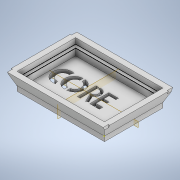
# Autodesk Inventor part: Rack holder aluminium
Saved by Autodesk Inventor 2021 (Build 250183000, 183)
## iProperties
Created: 2021-05-21
Part Number: Rack holder aluminium
Material: Generic
Document SubType Name: Modeling
Designer: Olivi
Density: 1 g/cm^3
Appearance: Default
Author: Olivi
Autodesk Inventor part; units mm, degrees
ref_plane "YZ Plane" through (0, 0, 0) normal (1, 0, 0) x (0, 1, 0)
ref_plane "XZ Plane" through (0, 0, 0) normal (0, 1, 0) x (-1, 0, 0)
ref_plane "XY Plane" through (0, 0, 0) normal (0, 0, 1) x (1, 0, 0)
sketch "Sketch1" plane through (0, 0, 0) normal (0, 1, 0) x (-1, 0, 0)
  line L0 (0, 0) -> (0, -85.5)
  line L1 (0, -85.5) -> (127.8, -85.5)
  line L2 (127.8, -85.5) -> (127.8, 0)
  line L3 (127.8, 0) -> (0, 0)
  dimension "d0" = 85.5
  dimension "d1" = 127.8
  constraints: 8 end point, 3 perpendicular, 1 vertical
  measures "d0" distance of L0.start L0.end
  measures "d1" distance of L0.end L1.end
extrude "Extrusion2" add sketch "Sketch1" along normal blind 7
sketch "Sketch3" plane through (0, 7, 0) normal (0, 1, 0) x (1, 0, 0)
  point P0 (0, 0)
sketch "Sketch4" plane through (0, 7, 0) normal (0, 1, 0) x (1, 0, 0)
  arc A0 (-101.824, 57.4968) -> (-102.1452, 30.5151) centre (-105.5468, 44.0484) ccw
  arc A1 (-103.7513, 52.0362) -> (-103.7513, 35.012) centre (-104.5875, 43.5241) ccw
  line L0 (-103.7513, 52.0362) -> (-101.824, 57.4968)
  line L1 (-103.7513, 35.012) -> (-102.1452, 30.5151)
  arc A2 (-88.634, 52.8416) -> (-88.8908, 35.2488) centre (-87.1081, 44.021) ccw
  arc A3 (-85.3254, 35.2488) -> (-85.5822, 52.8416) centre (-87.1081, 44.021) ccw
  arc A4 (-85.5822, 30.5151) -> (-85.5822, 57.4968) centre (-86.7037, 44.006) ccw
  line L2 (-85.5822, 57.4968) -> (-85.5822, 52.8416)
  line L3 (-85.3254, 35.2488) -> (-85.5822, 30.5151)
  line L4 (-88.8908, 35.2488) -> (-88.8908, 30.2611)
  line L5 (-88.634, 57.4969) -> (-88.634, 52.8416)
  arc A5 (-88.634, 57.4969) -> (-88.8908, 30.2611) centre (-88.5011, 43.8765) ccw
  line L6 (-69.8, 57.4969) -> (-69.8, 30.2611)
  line L7 (-69.8, 30.2611) -> (-65.8, 30.2611)
  line L8 (-65.8, 30.2611) -> (-65.8, 57.4969)
  line L9 (-65.8, 57.4969) -> (-69.8, 57.4969)
  line L10 (-57.9844, 30.2611) -> (-64.357, 43.879)
  arc A6 (-64.357, 43.879) -> (-64.357, 55.1692) centre (-63.6585, 49.5241) ccw
  line L11 (-57.9844, 30.2611) -> (-54.5512, 31.8677)
  line L12 (-54.5512, 31.8677) -> (-59.1663, 41.7297)
  arc A7 (-59.1663, 41.7297) -> (-64.357, 57.4969) centre (-62.8, 49.2714) ccw
  line L13 (-64.357, 57.4969) -> (-64.357, 55.1692)
  line L14 (-51.8, 58.0868) -> (-51.8, 30.2611)
  line L15 (-51.8, 30.2611) -> (-37.8, 30.2611)
  line L16 (-37.8, 30.2611) -> (-37.8, 35.2488)
  line L17 (-37.8, 35.2488) -> (-47.8, 35.2488)
  line L18 (-47.8, 35.2488) -> (-47.8, 43.5)
  line L19 (-47.8, 43.5) -> (-39.7884, 43.5)
  line L20 (-39.7884, 43.5) -> (-39.7884, 46.5)
  line L21 (-39.7884, 46.5) -> (-47.8, 46.5)
  line L22 (-47.8, 46.5) -> (-47.8, 54.5)
  line L23 (-47.8, 54.5) -> (-37.8, 54.5)
  line L24 (-37.8, 54.5) -> (-37.8, 58.0868)
  line L25 (-37.8, 58.0868) -> (-51.8, 58.0868)
  line L26 (-127.8, 85.5) -> (-127.8, 0) projected
  line L27 (0, 85.5) -> (-127.8, 85.5) projected
  point P0 (0, 0)
  dimension "d28" = 62
  dimension "d29" = 65
  dimension "d30" = 76
  dimension "d31" = 80
  dimension "d32" = 90
  dimension "d35" = 27.4132
  dimension "d36" = 31
  dimension "d37" = 39
  dimension "d38" = 42
  dimension "d39" = 50.2512
  dimension "d40" = 22.2532
  dimension "d43" = 58
  constraints: 52 end point, 19 point on circle, 13 perpendicular, 8 centre point, 6 vertical, 5 point on line, 1 concentric
  measures "d28" distance between parallel lines of L26 L8
  measures "d29" distance from line of L26 A7.centre
  measures "d30" distance between parallel lines of L26 L14
  measures "d31" distance between parallel lines of L26 L22
  measures "d32" distance between parallel lines of L26 L24
  measures "d35" distance between parallel lines of L27 L25
  measures "d36" distance between parallel lines of L23 L27
  measures "d37" distance between parallel lines of L21 L27
  measures "d38" distance between parallel lines of L27 L19
  measures "d39" distance between parallel lines of L17 L27
  measures "d40" distance from line of L26 A0.centre
  measures "d43" distance between parallel lines of L26 L6
extrude "Extrusion3" cut sketch "Sketch4" against normal through all
sketch "Sketch5" plane through (0, 7, 0) normal (0, 1, 0) x (1, 0, 0)
  line L0 (-127.8, 0) -> (0, 0) projected
  line L1 (-127.8, 0) -> (0, 0)
  line L2 (0, 0) -> (0, 85.5) projected
  line L3 (0, 0) -> (0, 85.5)
  line L4 (0, 85.5) -> (-127.8, 85.5) projected
  line L5 (0, 85.5) -> (-127.8, 85.5)
  line L6 (-127.8, 85.5) -> (-127.8, 0)
  line L7 (-122.8, 80.5) -> (-5, 80.5)
  line L8 (-5, 80.5) -> (-5, 4.1226)
  line L9 (-5, 4.1226) -> (-122.8, 4.1226)
  line L10 (-122.8, 4.1226) -> (-122.8, 80.5)
  line L11 (-127.8, 85.5) -> (-127.8, 0) projected
  dimension "d44" = 5
  dimension "d45" = 5
  dimension "d46" = 5
  constraints: 16 end point, 5 perpendicular, 3 equal length
  measures "d44" distance between parallel lines of L2 L8
  measures "d45" distance between parallel lines of L6 L10
  measures "d46" distance between parallel lines of L4 L7
extrude "Extrusion4" add sketch "Sketch5" along normal blind 10
sketch "Sketch9" plane through (0, 17, 0) normal (0, 1, 0) x (1, 0, 0)
  line L0 (-127.8, 85.5) -> (-127.8, 0) projected
  line L1 (-127.8, 0) -> (-127.8, 85.5)
  line L2 (-127.8, 85.5) -> (0, 85.5)
  line L3 (0, 85.5) -> (0, 0)
  line L4 (0, 0) -> (-127.8, 0)
  line L5 (-122.8, 4.1226) -> (-5, 4.1226) projected
  line L6 (-5, 80.5) -> (-122.8, 80.5) projected
  line L7 (-122.8, 4.1226) -> (-122.8, 80.5)
  line L8 (-122.8, 80.5) -> (-5, 80.5)
  line L9 (-5, 80.5) -> (-5, 4.1226)
  line L10 (-5, 4.1226) -> (-122.8, 4.1226)
  point P0 (0, 0)
  constraints: 16 end point, 5 equal length, 3 perpendicular
ref_plane "Work Plane4" through (-63.9, 0, 0) normal (1, 0, 0) x (0, 0, -1)
sketch "Sketch21" plane through (-63.9, 0, 0) normal (1, 0, 0) x (0, 0, -1)
  line L0 (0, 0) -> (0, 17) projected
  line L1 (0, 7.0438) -> (0, 25.0438)
  line L2 (0, 25.0438) -> (-8, 25.0438)
  line L3 (-8, 25.0438) -> (0, 7.0438)
  line L4 (85.5, 0) -> (85.5, 17) projected
  line L5 (85.5, 7.0438) -> (85.5, 25.0438)
  line L6 (85.5, 25.0438) -> (93.5, 25.0438)
  line L7 (93.5, 25.0438) -> (85.5, 7.0438)
  dimension "d99" = 18
  dimension "d100" = 8
  dimension "d101" = 18
  dimension "d102" = 8
  constraints: 12 end point, 2 collinear, 2 perpendicular, 2 point on line
  measures "d99" distance of L1.start L1.end
  measures "d100" distance of L1.end L2.end
  measures "d101" distance of L5.start L5.end
  measures "d102" distance of L5.end L6.end
extrude "Extrusion7" add sketch "Sketch21" along normal mid plane 140
ref_plane "Work Plane5" through (-127.8, 0, -42.7) normal (0, 0, 1) x (1, 0, 0)
sketch "Sketch22" plane through (-127.8, 0, -42.7) normal (0, 0, 1) x (1, 0, 0)
  line L0 (127.8, 7.0438) -> (133.9, 7.0438) projected
  line L1 (127.8, 7.0438) -> (127.8, 25.0438)
  line L2 (133.9, 25.0438) -> (-6.1, 25.0438) projected
  line L3 (127.8, 25.0438) -> (135.8, 25.0438)
  line L4 (135.8, 25.0438) -> (127.8, 7.0438)
  line L5 (0, 0) -> (0, 7.0438) projected
  line L6 (0, 7.0438) -> (0, 25.0438)
  line L7 (0, 25.0438) -> (-8, 25.0438)
  line L8 (-6.1, 7.0438) -> (0, 7.0438) projected
  line L9 (-8, 25.0438) -> (0, 7.0438)
  point P0 (127.8, 0)
  dimension "d106" = 8
  dimension "d107" = 8
  constraints: 12 end point, 3 point on line, 2 perpendicular, 1 vertical
  measures "d106" distance of L1.end L3.end
  measures "d107" distance of L6.end L7.end
extrude "Extrusion8" add sketch "Sketch22" along normal mid plane 86
sketch "Sketch24" plane through (-127.8, 0, 0) normal (0, 0, 1) x (1, 0, 0)
  line L0 (-6.1, 7.0438) -> (-6.1, 25.0438) projected
  line L1 (0, 7.0438) -> (127.8, 7.0438) projected
  line L2 (-6.1, 20.9849) -> (0, 7.0438)
  line L3 (0, 7.0438) -> (-6.1, 7.0438)
  line L4 (-6.1, 7.0438) -> (-6.1, 20.9849)
  line L5 (127.8, 7.0438) -> (133.9, 7.0438) projected
  line L6 (133.9, 7.0438) -> (133.9, 20.7688) projected
  line L7 (127.8, 7.0438) -> (133.9, 20.7688)
  line L8 (133.9, 20.7688) -> (133.9, 7.0438)
  line L9 (133.9, 7.0438) -> (127.8, 7.0438)
  point P0 (127.8, 0)
  constraints: 12 end point, 2 collinear, 2 perpendicular, 1 point on line
extrude "Extrusion9" cut sketch "Sketch24" along normal blind 86
sketch "Sketch25" plane through (0, 0, -85.5) normal (0, 0, -1) x (-1, 0, 0)
  line L0 (-6.1, 20.7688) -> (0, 7.0438) projected
  line L1 (0, 7.0438) -> (-6.1, 20.7688)
  line L2 (-6.1, 20.7688) -> (-6.1, 7.0438)
  line L3 (-6.1, 7.0438) -> (0, 7.0438)
  line L4 (127.8, 7.0438) -> (133.9, 20.7688) projected
  line L5 (127.8, 7.0438) -> (133.9, 20.7688)
  line L6 (133.9, 7.0438) -> (133.9, 20.7688) projected
  line L7 (133.9, 20.7688) -> (133.9, 7.0438)
  line L8 (127.8, 7.0438) -> (0, 7.0438) projected
  line L9 (133.9, 7.0438) -> (127.8, 7.0438)
  point P0 (0, 0)
  constraints: 12 end point, 3 collinear, 2 perpendicular, 1 point on line, 1 vertical
extrude "Extrusion10" cut sketch "Sketch25" along normal blind 86
body "Solid2"
